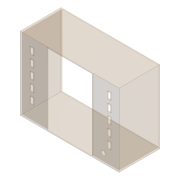
# Autodesk Inventor part: Board_Final_Concept
Saved by Autodesk Inventor 2012 (Build 160160000, 160)
## iProperties
Created: 2012-01-29
Part Number: Board_Final_Concept
Material: Wood (Birch)
Document SubType Name: Modeling
Designer: JesseK
Density: 1.02861 g/cm^3
Mass: 3946.25 g
Surface Area: 12377.2 cm^2
Volume: 3836.48 cm^3
Author: JesseK
Autodesk Inventor part; units mm, degrees
ref_plane "YZ Plane" through (0, 0, 0) normal (1, 0, 0) x (0, 1, 0)
ref_plane "XZ Plane" through (0, 0, 0) normal (0, 1, 0) x (-1, 0, 0)
ref_plane "XY Plane" through (0, 0, 0) normal (0, 0, 1) x (1, 0, 0)
sketch "Sketch1" plane through (0, 0, 0) normal (0, 0, 1) x (1, 0, 0)
  line L0 (0, 0) -> (584.2, 0)
  line L1 (584.2, 0) -> (584.2, 431.8)
  line L2 (584.2, 431.8) -> (0, 431.8)
  line L3 (0, 431.8) -> (0, 0)
  line L4 (6.35, 6.35) -> (577.85, 6.35)
  line L5 (577.85, 6.35) -> (577.85, 425.45)
  line L6 (577.85, 425.45) -> (6.35, 425.45)
  line L7 (6.35, 425.45) -> (6.35, 6.35)
  dimension "d0" = 6.35
  dimension "d1" = 6.35
  dimension "d2" = 6.35
  dimension "d3" = 6.35
  dimension "d4" = 584.2
  dimension "d5" = 431.8
  constraints: 16 end point, 4 parallel, 2 horizontal, 2 perpendicular
  measures "d0" distance between parallel lines of L0 L4
  measures "d1" distance between parallel lines of L2 L6
  measures "d2" distance between parallel lines of L1 L5
  measures "d3" distance between parallel lines of L7 L3
  measures "d4" distance between parallel lines of L1 L3
  measures "d5" distance of L2.end L0.start
extrude "Extrusion1" add sketch "Sketch1" along normal blind 241.3
sketch "Sketch2" plane through (6.35, 6.35, 241.3) normal (1, 0, 0) x (0, 0, -1)
  line L0 (0, 0) -> (0, 419.1) projected
  line L1 (241.3, 0) -> (0, 0) projected
  line L2 (0, 419.1) -> (6.35, 419.1)
  line L3 (6.35, 419.1) -> (6.35, 0)
  line L4 (6.35, 0) -> (0, 0)
  line L5 (0, 0) -> (0, 419.1)
  point P0 (241.3, -6.35)
  dimension "d8" = 6.35
  constraints: 8 end point, 2 parallel, 1 horizontal, 1 perpendicular, 1 point on line
  measures "d8" distance between parallel lines of L3 L5
extrude "Extrusion2" add sketch "Sketch2" along normal blind 152.4
sketch "Sketch3" plane through (577.85, 6.35, 241.3) normal (-1, 0, 0) x (0, 0, 1)
  line L0 (0, 419.1) -> (0, 0) projected
  line L1 (-241.3, 419.1) -> (0, 419.1) projected
  line L2 (0, 0) -> (-6.35, 0)
  line L3 (-6.35, 0) -> (-6.35, 419.1)
  line L4 (-6.35, 419.1) -> (0, 419.1)
  line L5 (0, 419.1) -> (0, 0)
  point P0 (-241.3, -6.35)
  dimension "d11" = 6.35
  constraints: 8 end point, 2 parallel, 1 horizontal, 1 perpendicular, 1 point on line
  measures "d11" distance between parallel lines of L5 L3
extrude "Extrusion3" add sketch "Sketch3" along normal blind 152.4
sketch "Sketch4" plane through (0, 0, 241.3) normal (0, 0, 1) x (1, 0, 0)
  line L0 (57.15, 381) -> (76.2, 381)
  line L1 (76.2, 381) -> (76.2, 342.9)
  line L2 (76.2, 342.9) -> (57.15, 342.9)
  line L3 (57.15, 342.9) -> (57.15, 381)
  line L4 (0, 0) -> (0, 431.8) projected
  line L5 (0, 431.8) -> (584.2, 431.8) projected
  dimension "d14" = 19.05
  dimension "d15" = 38.1
  dimension "d29" = 57.15
  dimension "d30" = 50.8
  constraints: 8 end point, 2 parallel, 1 horizontal, 1 perpendicular
  measures "d14" distance of L0.start L0.end
  measures "d15" distance of L2.end L0.start
  measures "d29" distance between parallel lines of L4 L3
  measures "d30" distance between parallel lines of L5 L0
extrude "Extrusion4" cut sketch "Sketch4" against normal up to next
pattern_linear "Rectangular Pattern1" count 5 spacing 63.5 along (0, -1, 0) count 2 spacing 457.2 along (1, 0, 0) of "Extrusion4"
sketch "Sketch5" plane through (0, 0, 241.3) normal (0, 0, 1) x (1, 0, 0)
  line L0 (425.45, 425.45) -> (425.45, 6.35) projected
  line L1 (584.2, 0) -> (0, 0) projected
  circle A0 centre (488.95, 50.8) radius 12.7
  dimension "d24" = 25.4
  dimension "d25" = 63.5
  dimension "d26" = 50.8
  constraints: 1 centre point
  measures "d24" diameter of A0
  measures "d25" distance from line of L0 A0.centre
  measures "d26" distance from line of L1 A0.centre
extrude "Extrusion5" cut sketch "Sketch5" against normal up to next
body "Solid1"
